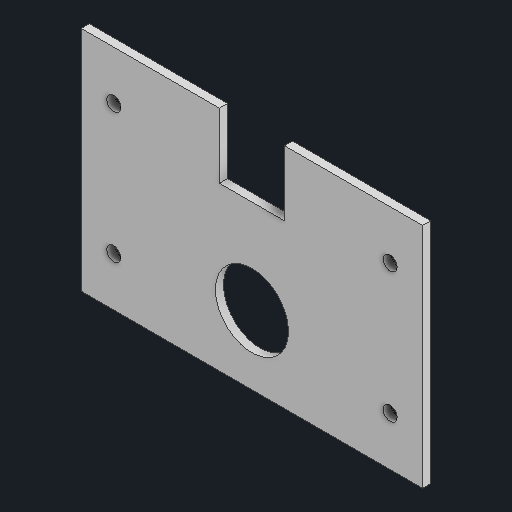
# Autodesk Inventor part: DIFF_PLATE_ROD_SHORT
Saved by Autodesk Inventor 2026.1 (Build 301233020, 233B)
## iProperties
Created: 2024-01-10
Part Number: DIFF_PLATE_ROD_SHORT
Material: Generic
Document SubType Name: Modeling
Designer: bugme
Density: 1 g/cm^3
Appearance: Default
Author: bugme
Autodesk Inventor part; units mm, degrees
ref_plane "YZ Plane" through (0, 0, 0) normal (1, 0, 0) x (0, 1, 0)
ref_plane "XZ Plane" through (0, 0, 0) normal (0, 1, 0) x (-1, 0, 0)
ref_plane "XY Plane" through (0, 0, 0) normal (0, 0, 1) x (1, 0, 0)
sketch "Sketch1" plane through (0, 0, 0) normal (0, 0, 1) x (1, 0, 0)
  line L0 (0, -17.78) -> (0, 106.68) projected
  line L1 (66.675, 88.9) -> (66.675, 0)
  line L2 (66.675, 0) -> (-66.675, 0)
  line L3 (-66.675, 0) -> (-66.675, 88.9)
  line L4 (-93.345, 0) -> (93.345, 0) projected
  line L5 (-12.7, 88.9) -> (-12.7, 63.5)
  line L6 (-12.7, 63.5) -> (12.7, 63.5)
  line L7 (12.7, 63.5) -> (12.7, 88.9)
  line L8 (-66.675, 88.9) -> (-12.7, 88.9)
  line L9 (12.7, 88.9) -> (66.675, 88.9)
  line L10 (0, 0) -> (0, 26.797)
  circle A0 centre (0, 26.797) radius 14.2875
  dimension "d0" = 133.35
  dimension "d1" = 88.9
  dimension "d2" = 25.4
  dimension "d3" = 25.4
  dimension "d5" = 28.575
  dimension "d19" = 62.103
  constraints: 18 end point, 4 perpendicular, 2 horizontal, 2 midpoint, 2 vertical, 1 centre point, 1 coincident, 1 point on line, 1 symmetric about line, 1 other
  measures "d0" distance of L3.end L1.start
  measures "d1" distance of L1.start L1.end
  measures "d2" distance of L5.start L5.end
  measures "d3" distance of L5.end L6.end
  measures "d5" diameter of A0
  measures "d19" distance from line of A0.centre L8
extrude "Extrusion1" add sketch "Sketch1" along normal blind 3.175 contours L2 L3 L8 L5 L6 L0 A0 | L0 A0 L6 L7 L9 L1 L2
sketch "Sketch2" plane through (0, 0, 3.175) normal (0, 0, 1) x (1, 0, 0)
  line L0 (66.675, 0) -> (66.675, 88.9) projected
  line L1 (-66.675, 0) -> (66.675, 0) projected
  line L2 (66.675, 88.9) -> (12.7, 88.9) projected
  point P0 (0, 0)
  point P1 (53.975, 69.85)
  point P2 (53.975, 19.05)
  dimension "d16" = 12.7
  dimension "d18" = 19.05
  dimension "d20" = 19.05
  constraints: 1 vertical alignment
  measures "d16" distance from line of L0 point (53.975, 69.85)
  measures "d18" distance from line of L1 point (53.975, 19.05)
  measures "d20" distance from line of L2 point (53.975, 69.85)
hole "Hole1" at (53.975, 69.85, 3.175) at (53.975, 19.05, 3.175) direction (0, 0, -1) diameter 5.5118 end through all clearance for "Flat Head Machine Screw" size "M5" standard "Ansi Metric M Profile"
mirror "Mirror1" about plane through (0, 0, 0) normal (1, 0, 0) of "Hole1"
equation "\"d20\" = d18"
body "Solid1"
